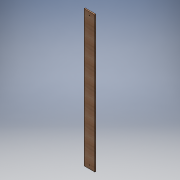
# Autodesk Inventor part: spielfeld_trennwand
Saved by Autodesk Inventor 2016 SP2 (Build 200236200, 236)
## iProperties
Created: 2018-04-09
Part Number: spielfeld_trennwand
Material: Spanplatte
Document SubType Name: Modeling
Designer: wepet
Density: 1 g/cm^3
Appearance: Birke - natur- poliert
Mass: 5118.39 g
Surface Area: 7097.23 cm^2
Volume: 5118.39 cm^3
Author: wepet
Autodesk Inventor part; units mm, degrees
ref_plane "YZ Plane" through (0, 0, 0) normal (1, 0, 0) x (0, 1, 0)
ref_plane "XZ Plane" through (0, 0, 0) normal (0, 1, 0) x (-1, 0, 0)
ref_plane "XY Plane" through (0, 0, 0) normal (0, 0, 1) x (1, 0, 0)
sketch "Skizze1" plane through (0, 0, 0) normal (0, 1, 0) x (-1, 0, 0)
  line L0 (0, 0) -> (160, 0)
  line L1 (160, 0) -> (160, -2000)
  line L2 (160, -2000) -> (0, -2000)
  line L3 (0, -2000) -> (0, 0)
  dimension "d0" = 160
  dimension "d1" = 2000
  constraints: 8 end point, 2 parallel, 1 horizontal, 1 perpendicular
  measures "d0" distance of L1.end L2.end
  measures "d1" distance of L0.end L1.end
extrude "Extrusion1" add sketch "Skizze1" along normal blind 16
sketch "Skizze2" plane through (0, 16, 0) normal (0, 1, 0) x (1, 0, 0)
  line L0 (-160, 0) -> (0, 0) projected
  line L1 (0, 0) -> (0, 2000) projected
  line L2 (0, 2000) -> (-160, 2000) projected
  line L3 (-160, 2000) -> (-160, 0) projected
  point P0 (-80, 50)
  point P1 (-80, 1950)
  dimension "d4" = 80
  dimension "d5" = 50
  dimension "d6" = 50
  dimension "d7" = 80
  measures "d4" distance from line of L1 point (-80, 50)
  measures "d5" distance from line of L0 point (-80, 50)
  measures "d6" distance from line of L2 point (-80, 1950)
  measures "d7" distance from line of L1 point (-80, 1950)
hole "Bohrung1" at (-80, 16, -50) at (-80, 16, -1950) direction (0, -1, 0) diameter 8 end through all
